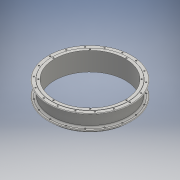
# Autodesk Inventor part: Pièce1
Saved by Autodesk Inventor 2016 (Build 200138000, 138)
## iProperties
Created: 2015-11-15
Part Number: Pièce1
Material: Générique
Document SubType Name: Modeling
Designer: Cyril
Density: 1 g/cm^3
Appearance: Par défaut
Author: Cyril
Autodesk Inventor part; units mm, degrees
ref_plane "YZ Plane" through (0, 0, 0) normal (1, 0, 0) x (0, 1, 0)
ref_plane "XZ Plane" through (0, 0, 0) normal (0, 1, 0) x (-1, 0, 0)
ref_plane "XY Plane" through (0, 0, 0) normal (0, 0, 1) x (1, 0, 0)
sketch "Esquisse1" plane through (0, 0, 0) normal (1, 0, 0) x (0, 1, 0)
  line L0 (0, 0) -> (115, 0) construction
  line L1 (115, 0) -> (115, 15.5)
  arc A0 (120, 20.5) -> (115, 15.5) centre (120, 15.5) ccw
  line L2 (120, 20.5) -> (125, 20.5)
  arc A1 (125, 20.5) -> (125, 23.5) centre (125, 22) ccw
  line L3 (115, 0) -> (115, -15.5)
  arc A2 (115, -15.5) -> (120, -20.5) centre (120, -15.5) ccw
  line L4 (120, -20.5) -> (125, -20.5)
  arc A3 (125, -23.5) -> (125, -20.5) centre (125, -22) ccw
  line L5 (125, 23.5) -> (115.5, 23.5)
  arc A4 (115, 24) -> (115.5, 23.5) centre (115.5, 24) ccw
  line L6 (115, 24) -> (106.5, 24)
  arc A5 (117, -23.5) -> (115, -25.5) centre (117, -25.5) ccw
  line L7 (117, -23.5) -> (125, -23.5)
  line L8 (115, -25.5) -> (115, -32.5)
  line L9 (115, -32.5) -> (106.5, -32.5)
  line L10 (106.5, 24) -> (106.5, -32.5)
  line L11 (0, 24) -> (0, -32.5) construction
  dimension "d0" = 1.5
  dimension "d1" = 5
  dimension "d2" = 2
  dimension "d3" = 0.5
  dimension "d27" = 125
  dimension "d28" = 115
  dimension "d29" = 47
  dimension "d30" = 106.5
  dimension "d31" = 56.5
  constraints: 24 end point, 12 point on circle, 7 tangent, 6 centre point, 6 horizontal, 6 point on line, 6 symmetric about line, 4 vertical, 2 other
  measures "d0" radius of A1
  measures "d1" radius of A0
  measures "d2" radius of A5
  measures "d3" radius of A4
  measures "d27" horizontal distance of L0.start A1.centre
  measures "d28" horizontal distance of L0.start L6.start
  measures "d29" distance between parallel lines of L7 L5
  measures "d30" distance between parallel lines of L11 L10
  measures "d31" distance between parallel lines of L9 L6
revolve "Révolution1" add sketch "Esquisse1" angle 360 about axis through (0, 0, 24) along (0, 0, -1)
sketch "Esquisse2" plane through (0, 0, 23.5) normal (0, 0, 1) x (1, 0, 0)
  circle A0 centre (-120, 0) radius 2.1
  circle A1 centre (-112.7631, -41.0424) radius 2.1
  circle A2 centre (-91.9253, -77.1345) radius 2.1
  circle A3 centre (-60, -103.923) radius 2.1
  circle A4 centre (-20.8378, -118.1769) radius 2.1
  circle A5 centre (20.8378, -118.1769) radius 2.1
  circle A6 centre (60, -103.923) radius 2.1
  circle A7 centre (91.9253, -77.1345) radius 2.1
  circle A8 centre (112.7631, -41.0424) radius 2.1
  circle A9 centre (120, 0) radius 2.1
  circle A10 centre (112.7631, 41.0424) radius 2.1
  circle A11 centre (91.9253, 77.1345) radius 2.1
  circle A12 centre (60, 103.923) radius 2.1
  circle A13 centre (20.8378, 118.1769) radius 2.1
  circle A14 centre (-20.8378, 118.1769) radius 2.1
  circle A15 centre (-60, 103.923) radius 2.1
  circle A16 centre (-91.9253, 77.1345) radius 2.1
  circle A17 centre (-112.7631, 41.0424) radius 2.1
  line L0 (-120, 0) -> (120, 0) construction
  point P0 (0, 0)
  dimension "d9" = 4.2
  dimension "d12" = 360
  dimension "d14" = 240
  constraints: 18 centre point, 2 end point, 1 horizontal, 37 other
  measures "d9" diameter of A0
  measures "d14" distance of L0.start L0.end
extrude "Extrusion1" cut sketch "Esquisse2" against normal blind 15
sketch "Esquisse3" plane through (0, 0, -23.5) normal (0, 0, -1) x (-1, 0, 0)
  circle A0 centre (0, 120) radius 2.1
  line L0 (0, 0) -> (0, 120) construction
  circle A1 centre (-41.0424, 112.7631) radius 2.1
  circle A2 centre (-77.1345, 91.9253) radius 2.1
  circle A3 centre (-103.923, 60) radius 2.1
  circle A4 centre (-118.1769, 20.8378) radius 2.1
  circle A5 centre (-118.1769, -20.8378) radius 2.1
  circle A6 centre (-103.923, -60) radius 2.1
  circle A7 centre (-77.1345, -91.9253) radius 2.1
  circle A8 centre (-41.0424, -112.7631) radius 2.1
  circle A9 centre (0, -120) radius 2.1
  circle A10 centre (41.0424, -112.7631) radius 2.1
  circle A11 centre (77.1345, -91.9253) radius 2.1
  circle A12 centre (103.923, -60) radius 2.1
  circle A13 centre (118.1769, -20.8378) radius 2.1
  circle A14 centre (118.1769, 20.8378) radius 2.1
  circle A15 centre (103.923, 60) radius 2.1
  circle A16 centre (77.1345, 91.9253) radius 2.1
  circle A17 centre (41.0424, 112.7631) radius 2.1
  dimension "d19" = 4.2
  dimension "d22" = 360
  dimension "d24" = 240
  constraints: 18 centre point, 2 end point, 1 vertical, 37 other
  measures "d19" diameter of A0
  measures "d24" distance of A9.centre L0.end
extrude "Extrusion2" cut sketch "Esquisse3" against normal blind 10
sketch "Esquisse4" plane through (0, 0, 24) normal (0, 0, 1) x (1, 0, 0)
  line L0 (0, -177.1) -> (0, 177.1) projected
  point P0 (0, 0)
  point P1 (0, 110)
  point P2 (-77.7817, 77.7817)
  point P3 (-110, 0)
  point P4 (-77.7817, -77.7817)
  point P5 (0, -110)
  point P6 (77.7817, -77.7817)
  point P7 (110, 0)
  point P8 (77.7817, 77.7817)
  dimension "d34" = 360
  dimension "d36" = 220
  constraints: 1 point on line, 9 other
  measures "d36" distance of point (0, -110) point (0, 110)
hole "Perçage1" at (0, 110, 24) at (-77.7817, 77.7817, 24) at (-110, 0, 24) at (-77.7817, -77.7817, 24) at (0, -110, 24) at (77.7817, -77.7817, 24) at (110, 0, 24) at (77.7817, 77.7817, 24) direction (0, 0, -1) diameter 4.134 depth 14 tip angle 118 thread size "M5x0.8" class "6H" standard "ISO Metric profile"
sketch "Esquisse5" plane through (0, 0, -32.5) normal (0, 0, -1) x (-1, 0, 0)
  line L0 (0, 0) -> (0, 110) construction
  point P0 (-77.7817, 77.7817)
  point P1 (-110, 0)
  point P2 (-77.7817, -77.7817)
  point P3 (0, -110)
  point P4 (77.7817, -77.7817)
  point P5 (110, 0)
  point P6 (77.7817, 77.7817)
  dimension "d46" = 360
  dimension "d48" = 220
  constraints: 2 end point, 1 vertical, 9 other
  measures "d48" distance of point (0, -110) L0.end
hole "Perçage2" at (0, 110, -32.5) at (77.7817, 77.7817, -32.5) at (110, 0, -32.5) at (77.7817, -77.7817, -32.5) at (0, -110, -32.5) at (-77.7817, -77.7817, -32.5) at (-110, 0, -32.5) at (-77.7817, 77.7817, -32.5) direction (0, 0, 1) diameter 4.134 depth 14 tip angle 118 thread size "M5x0.8" class "6H" standard "ISO Metric profile"
